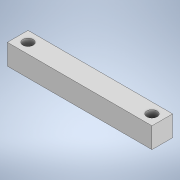
# Autodesk Inventor part: short_link_v1
Saved by Autodesk Inventor 2022 (Build 260153000, 153)
## iProperties
Created: 2022-05-21
Part Number: short_link_v1
Material: Generic
Document SubType Name: Modeling
Designer: kylem
Density: 1 g/cm^3
Appearance: Default
Author: kylem
Autodesk Inventor part; units mm, degrees
ref_plane "YZ Plane" through (0, 0, 0) normal (1, 0, 0) x (0, 1, 0)
ref_plane "XZ Plane" through (0, 0, 0) normal (0, 1, 0) x (-1, 0, 0)
ref_plane "XY Plane" through (0, 0, 0) normal (0, 0, 1) x (1, 0, 0)
sketch "Sketch1" plane through (0, 0, 0) normal (0, 1, 0) x (-1, 0, 0)
  line L0 (0, 0) -> (14, 0)
  line L1 (14, 0) -> (14, -2)
  line L2 (14, -2) -> (0, -2)
  line L3 (0, -2) -> (0, 0)
  line L4 (14, -1) -> (13, -1)
  line L5 (7, -2) -> (7, -1)
  circle A0 centre (13, -1) radius 0.5
  circle A1 centre (1, -1) radius 0.5
  dimension "d0" = 14
  dimension "d1" = 2
  dimension "d2" = 1
  dimension "d3" = 1
  constraints: 12 end point, 2 centre point, 2 horizontal, 2 midpoint, 2 parallel, 1 coincident, 1 perpendicular, 1 symmetric about line, 1 vertical, 1 other
  measures "d0" distance of L1.end L2.end
  measures "d1" distance of L0.end L1.end
  measures "d2" distance of L4.start L4.end
  measures "d3" diameter of A0
extrude "Extrusion1" add sketch "Sketch1" along normal blind 2
body "Solid1"
